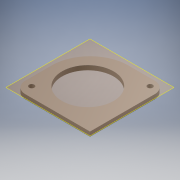
# Autodesk Inventor part: base
Saved by Autodesk Inventor 2016 (Build 200138000, 138)
## iProperties
Created: 2016-01-18
Part Number: base
Material: Generic
Document SubType Name: Modeling
Designer: Erwin Ried
Density: 1 g/cm^3
Appearance: Default
Author: Erwin Ried
Autodesk Inventor part; units mm, degrees
ref_plane "YZ Plane" through (0, 0, 0) normal (1, 0, 0) x (0, 1, 0)
ref_plane "XZ Plane" through (0, 0, 0) normal (0, 1, 0) x (-1, 0, 0)
ref_plane "XY Plane" through (0, 0, 0) normal (0, 0, 1) x (1, 0, 0)
ref_plane "Work Plane1" through (0, 0, 0) normal (0, 0, 1) x (1, 0, 0)
sketch "Sketch1" plane through (0, 0, 0) normal (0, 0, 1) x (1, 0, 0)
  line L0 (-5.1606, -11.1286) -> (-4.5083, -12.1241) projected
  line L1 (-4.5083, -12.1241) -> (-3.9263, -13.1603) projected
  line L2 (-3.9263, -13.1603) -> (-3.4128, -14.2404) projected
  line L3 (-3.4128, -14.2404) -> (-2.9734, -15.3534) projected
  line L4 (-2.9734, -15.3534) -> (-2.6124, -16.4922) projected
  line L5 (-2.6124, -16.4922) -> (-2.3286, -17.6568) projected
  line L6 (-2.3286, -17.6568) -> (-2.126, -18.8312) projected
  line L7 (-2.126, -18.8312) -> (-2.0043, -20.0161) projected
  line L8 (-2.0043, -20.0161) -> (-1.9632, -21.2132) projected
  line L9 (-2.0053, -22.4191) -> (-1.9632, -21.2132) projected
  line L10 (-2.1283, -23.6107) -> (-2.0053, -22.4191) projected
  line L11 (-2.3328, -24.7898) -> (-2.1283, -23.6107) projected
  line L12 (-2.6189, -25.957) -> (-2.3328, -24.7898) projected
  line L13 (-2.9818, -27.0966) -> (-2.6189, -25.957) projected
  line L14 (-3.4226, -28.2085) -> (-2.9818, -27.0966) projected
  line L15 (-3.9367, -29.2861) -> (-3.4226, -28.2085) projected
  line L16 (-4.5183, -30.3188) -> (-3.9367, -29.2861) projected
  line L17 (-5.169, -31.3097) -> (-4.5183, -30.3188) projected
  line L18 (-5.8865, -32.2545) -> (-5.169, -31.3097) projected
  line L19 (-6.6737, -33.1569) -> (-5.8865, -32.2545) projected
  line L20 (-7.5197, -34.0039) -> (-6.6737, -33.1569) projected
  line L21 (-8.4188, -34.7876) -> (-7.5197, -34.0039) projected
  line L22 (-9.3708, -35.5096) -> (-8.4188, -34.7876) projected
  line L23 (-10.3652, -36.1622) -> (-9.3708, -35.5096) projected
  line L24 (-11.405, -36.7472) -> (-10.3652, -36.1622) projected
  line L25 (-12.4791, -37.2591) -> (-11.405, -36.7472) projected
  line L26 (-13.5862, -37.6966) -> (-12.4791, -37.2591) projected
  line L27 (-14.722, -38.0586) -> (-13.5862, -37.6966) projected
  line L28 (-15.8764, -38.3415) -> (-14.722, -38.0586) projected
  line L29 (-17.0521, -38.5461) -> (-15.8764, -38.3415) projected
  line L30 (-18.2354, -38.67) -> (-17.0521, -38.5461) projected
  line L31 (-19.4276, -38.7129) -> (-18.2354, -38.67) projected
  line L32 (-20.6207, -38.6749) -> (-19.4276, -38.7129) projected
  line L33 (-21.8064, -38.5553) -> (-20.6207, -38.6749) projected
  line L34 (-22.9861, -38.3548) -> (-21.8064, -38.5553) projected
  line L35 (-24.1458, -38.0749) -> (-22.9861, -38.3548) projected
  line L36 (-25.2885, -37.7149) -> (-24.1458, -38.0749) projected
  line L37 (-26.4032, -37.2782) -> (-25.2885, -37.7149) projected
  line L38 (-27.4856, -36.7657) -> (-26.4032, -37.2782) projected
  line L39 (-28.534, -36.1787) -> (-27.4856, -36.7657) projected
  line L40 (-29.5366, -35.523) -> (-28.534, -36.1787) projected
  line L41 (-30.4963, -34.7966) -> (-29.5366, -35.523) projected
  line L42 (-31.4021, -34.0081) -> (-30.4963, -34.7966) projected
  line L43 (-32.2538, -33.1556) -> (-31.4021, -34.0081) projected
  line L44 (-33.0454, -32.2477) -> (-32.2538, -33.1556) projected
  line L45 (-33.7658, -31.2978) -> (-33.0454, -32.2477) projected
  line L46 (-34.4181, -30.3023) -> (-33.7658, -31.2978) projected
  line L47 (-35.0001, -29.2661) -> (-34.4181, -30.3023) projected
  line L48 (-35.5136, -28.186) -> (-35.0001, -29.2661) projected
  line L49 (-35.9529, -27.073) -> (-35.5136, -28.186) projected
  line L50 (-36.314, -25.9342) -> (-35.9529, -27.073) projected
  line L51 (-36.5978, -24.7695) -> (-36.314, -25.9342) projected
  line L52 (-36.8004, -23.5952) -> (-36.5978, -24.7695) projected
  line L53 (-36.9221, -22.4103) -> (-36.8004, -23.5952) projected
  line L54 (-36.9632, -21.2132) -> (-36.9221, -22.4103) projected
  line L55 (-36.9632, -21.2132) -> (-36.9211, -20.0072) projected
  line L56 (-36.9211, -20.0072) -> (-36.7981, -18.8157) projected
  line L57 (-36.7981, -18.8157) -> (-36.5936, -17.6366) projected
  line L58 (-36.5936, -17.6366) -> (-36.3075, -16.4694) projected
  line L59 (-36.3075, -16.4694) -> (-35.9446, -15.3298) projected
  line L60 (-35.9446, -15.3298) -> (-35.5038, -14.2179) projected
  line L61 (-35.5038, -14.2179) -> (-34.9897, -13.1403) projected
  line L62 (-34.9897, -13.1403) -> (-34.4081, -12.1076) projected
  line L63 (-34.4081, -12.1076) -> (-33.7574, -11.1167) projected
  line L64 (-33.7574, -11.1167) -> (-33.0399, -10.1719) projected
  line L65 (-33.0399, -10.1719) -> (-32.2527, -9.2695) projected
  line L66 (-32.2527, -9.2695) -> (-31.4066, -8.4225) projected
  line L67 (-31.4066, -8.4225) -> (-30.5076, -7.6388) projected
  line L68 (-30.5076, -7.6388) -> (-29.5556, -6.9168) projected
  line L69 (-29.5556, -6.9168) -> (-28.5612, -6.2641) projected
  line L70 (-28.5612, -6.2641) -> (-27.5214, -5.6792) projected
  line L71 (-27.5214, -5.6792) -> (-26.4473, -5.1673) projected
  line L72 (-26.4473, -5.1673) -> (-25.3402, -4.7298) projected
  line L73 (-25.3402, -4.7298) -> (-24.2044, -4.3678) projected
  line L74 (-24.2044, -4.3678) -> (-23.05, -4.0849) projected
  line L75 (-23.05, -4.0849) -> (-21.8743, -3.8803) projected
  line L76 (-21.8743, -3.8803) -> (-20.691, -3.7564) projected
  line L77 (-20.691, -3.7564) -> (-19.4988, -3.7135) projected
  line L78 (-19.4988, -3.7135) -> (-18.3057, -3.7515) projected
  line L79 (-18.3057, -3.7515) -> (-17.12, -3.8711) projected
  line L80 (-17.12, -3.8711) -> (-15.9403, -4.0716) projected
  line L81 (-15.9403, -4.0716) -> (-14.7806, -4.3515) projected
  line L82 (-14.7806, -4.3515) -> (-13.6379, -4.7115) projected
  line L83 (-13.6379, -4.7115) -> (-12.5232, -5.1482) projected
  line L84 (-12.5232, -5.1482) -> (-11.4408, -5.6607) projected
  line L85 (-11.4408, -5.6607) -> (-10.3924, -6.2477) projected
  line L86 (-10.3924, -6.2477) -> (-9.3899, -6.9034) projected
  line L87 (-9.3899, -6.9034) -> (-8.4301, -7.6298) projected
  line L88 (-8.4301, -7.6298) -> (-7.5242, -8.4183) projected
  line L89 (-7.5242, -8.4183) -> (-6.6726, -9.2707) projected
  line L90 (-6.6726, -9.2707) -> (-5.881, -10.1787) projected
  line L91 (-5.881, -10.1787) -> (-5.1606, -11.1286) projected
  line L92 (-36.9509, -39.6064) -> (-36.8705, -39.831) projected
  line L93 (-36.8705, -39.831) -> (-36.8223, -40.0632) projected
  line L94 (-36.8223, -40.0632) -> (-36.8051, -40.3051) projected
  line L95 (-36.8222, -40.5477) -> (-36.8051, -40.3051) projected
  line L96 (-36.8711, -40.7811) -> (-36.8222, -40.5477) projected
  line L97 (-36.9527, -41.0075) -> (-36.8711, -40.7811) projected
  line L98 (-37.0645, -41.2218) -> (-36.9527, -41.0075) projected
  line L99 (-37.2034, -41.4163) -> (-37.0645, -41.2218) projected
  line L100 (-37.3681, -41.5909) -> (-37.2034, -41.4163) projected
  line L101 (-37.5533, -41.7398) -> (-37.3681, -41.5909) projected
  line L102 (-37.7583, -41.8631) -> (-37.5533, -41.7398) projected
  line L103 (-37.9764, -41.9564) -> (-37.7583, -41.8631) projected
  line L104 (-38.2075, -42.0201) -> (-37.9764, -41.9564) projected
  line L105 (-38.4425, -42.0513) -> (-38.2075, -42.0201) projected
  line L106 (-38.6818, -42.0504) -> (-38.4425, -42.0513) projected
  line L107 (-38.9165, -42.0171) -> (-38.6818, -42.0504) projected
  line L108 (-39.1474, -41.9514) -> (-38.9165, -42.0171) projected
  line L109 (-39.3645, -41.8566) -> (-39.1474, -41.9514) projected
  line L110 (-39.5677, -41.7322) -> (-39.3645, -41.8566) projected
  line L111 (-39.7505, -41.5831) -> (-39.5677, -41.7322) projected
  line L112 (-39.9126, -41.4092) -> (-39.7505, -41.5831) projected
  line L113 (-40.0492, -41.216) -> (-39.9126, -41.4092) projected
  line L114 (-40.1593, -41.0037) -> (-40.0492, -41.216) projected
  line L115 (-40.2396, -40.7792) -> (-40.1593, -41.0037) projected
  line L116 (-40.2879, -40.547) -> (-40.2396, -40.7792) projected
  line L117 (-40.3051, -40.3051) -> (-40.2879, -40.547) projected
  line L118 (-40.3051, -40.3051) -> (-40.2879, -40.0625) projected
  line L119 (-40.2879, -40.0625) -> (-40.2391, -39.8291) projected
  line L120 (-40.2391, -39.8291) -> (-40.1575, -39.6027) projected
  line L121 (-40.1575, -39.6027) -> (-40.0457, -39.3884) projected
  line L122 (-40.0457, -39.3884) -> (-39.9067, -39.1939) projected
  line L123 (-39.9067, -39.1939) -> (-39.742, -39.0192) projected
  line L124 (-39.742, -39.0192) -> (-39.5569, -38.8704) projected
  line L125 (-39.5569, -38.8704) -> (-39.3518, -38.7471) projected
  line L126 (-39.3518, -38.7471) -> (-39.1338, -38.6538) projected
  line L127 (-39.1338, -38.6538) -> (-38.9026, -38.5901) projected
  line L128 (-38.9026, -38.5901) -> (-38.6677, -38.5588) projected
  line L129 (-38.6677, -38.5588) -> (-38.4284, -38.5598) projected
  line L130 (-38.4284, -38.5598) -> (-38.1936, -38.593) projected
  line L131 (-38.1936, -38.593) -> (-37.9627, -38.6587) projected
  line L132 (-37.9627, -38.6587) -> (-37.7456, -38.7536) projected
  line L133 (-37.7456, -38.7536) -> (-37.5425, -38.878) projected
  line L134 (-37.5425, -38.878) -> (-37.3596, -39.0271) projected
  line L135 (-37.3596, -39.0271) -> (-37.1975, -39.2009) projected
  line L136 (-37.1975, -39.2009) -> (-37.0609, -39.3941) projected
  line L137 (-37.0609, -39.3941) -> (-36.9509, -39.6064) projected
  line L138 (-40.1775, -46.0183) -> (-39.5312, -46.3784) projected
  line L139 (-39.5312, -46.3784) -> (-38.8571, -46.6766) projected
  line L140 (-38.8571, -46.6766) -> (-38.1554, -46.9119) projected
  line L141 (-38.1554, -46.9119) -> (-37.4366, -47.0815) projected
  line L142 (-37.4366, -47.0815) -> (-36.7069, -47.1834) projected
  line L143 (-36.7069, -47.1834) -> (-35.9632, -47.2184) projected
  line L144 (-35.9632, -47.2184) -> (-11.9632, -47.2184) projected
  line L145 (-11.9632, -47.2184) -> (-10.4632, -47.2184) projected
  line L146 (-10.4632, -47.2184) -> (6.5368, -47.2184) projected
  line L147 (6.5368, -47.2184) -> (8.0368, -47.2184) projected
  line L148 (8.0368, -47.2184) -> (8.0368, -3.2184) projected
  line L149 (8.0018, -2.4748) -> (8.0368, -3.2184) projected
  line L150 (7.8999, -1.745) -> (8.0018, -2.4748) projected
  line L151 (7.7304, -1.0263) -> (7.8999, -1.745) projected
  line L152 (7.495, -0.3246) -> (7.7304, -1.0263) projected
  line L153 (7.1969, 0.3495) -> (7.495, -0.3246) projected
  line L154 (6.8367, 0.9958) -> (7.1969, 0.3495) projected
  line L155 (6.4204, 1.6031) -> (6.8367, 0.9958) projected
  line L156 (5.9478, 2.1721) -> (6.4204, 1.6031) projected
  line L157 (5.4274, 2.6925) -> (5.9478, 2.1721) projected
  line L158 (4.8584, 3.1651) -> (5.4274, 2.6925) projected
  line L159 (4.2511, 3.5814) -> (4.8584, 3.1651) projected
  line L160 (3.6048, 3.9416) -> (4.2511, 3.5814) projected
  line L161 (2.9307, 4.2397) -> (3.6048, 3.9416) projected
  line L162 (2.229, 4.4751) -> (2.9307, 4.2397) projected
  line L163 (1.5103, 4.6447) -> (2.229, 4.4751) projected
  line L164 (0.7805, 4.7466) -> (1.5103, 4.6447) projected
  line L165 (0.0368, 4.7816) -> (0.7805, 4.7466) projected
  line L166 (-17.9632, 4.7816) -> (0.0368, 4.7816) projected
  line L167 (-19.4279, 4.7399) -> (-17.9632, 4.7816) projected
  line L168 (-20.8805, 4.6173) -> (-19.4279, 4.7399) projected
  line L169 (-22.322, 4.4136) -> (-20.8805, 4.6173) projected
  line L170 (-23.7547, 4.1281) -> (-22.322, 4.4136) projected
  line L171 (-25.1672, 3.7636) -> (-23.7547, 4.1281) projected
  line L172 (-26.5555, 3.3206) -> (-25.1672, 3.7636) projected
  line L173 (-27.9196, 2.7995) -> (-26.5555, 3.3206) projected
  line L174 (-29.2482, 2.2048) -> (-27.9196, 2.7995) projected
  line L175 (-30.5443, 1.5347) -> (-29.2482, 2.2048) projected
  line L176 (-31.8002, 0.7938) -> (-30.5443, 1.5347) projected
  line L177 (-33.0104, -0.0153) -> (-31.8002, 0.7938) projected
  line L178 (-34.1764, -0.893) -> (-33.0104, -0.0153) projected
  line L179 (-35.2883, -1.8318) -> (-34.1764, -0.893) projected
  line L180 (-36.3477, -2.8337) -> (-35.2883, -1.8318) projected
  line L181 (-37.3497, -3.8932) -> (-36.3477, -2.8337) projected
  line L182 (-38.2885, -5.0051) -> (-37.3497, -3.8932) projected
  line L183 (-39.1662, -6.1711) -> (-38.2885, -5.0051) projected
  line L184 (-39.9753, -7.3813) -> (-39.1662, -6.1711) projected
  line L185 (-40.7162, -8.6371) -> (-39.9753, -7.3813) projected
  line L186 (-41.3863, -9.9332) -> (-40.7162, -8.6371) projected
  line L187 (-41.9811, -11.2619) -> (-41.3863, -9.9332) projected
  line L188 (-42.5022, -12.626) -> (-41.9811, -11.2619) projected
  line L189 (-42.9452, -14.0143) -> (-42.5022, -12.626) projected
  line L190 (-43.3097, -15.4268) -> (-42.9452, -14.0143) projected
  line L191 (-43.5951, -16.8595) -> (-43.3097, -15.4268) projected
  line L192 (-43.7989, -18.3011) -> (-43.5951, -16.8595) projected
  line L193 (-43.9215, -19.7537) -> (-43.7989, -18.3011) projected
  line L194 (-43.9632, -21.2184) -> (-43.9215, -19.7537) projected
  line L195 (-43.9632, -39.2184) -> (-43.9632, -21.2184) projected
  line L196 (-43.9632, -39.2184) -> (-43.9282, -39.962) projected
  line L197 (-43.9282, -39.962) -> (-43.8263, -40.6918) projected
  line L198 (-43.8263, -40.6918) -> (-43.6568, -41.4105) projected
  line L199 (-43.6568, -41.4105) -> (-43.4214, -42.1122) projected
  line L200 (-43.4214, -42.1122) -> (-43.1233, -42.7863) projected
  line L201 (-43.1233, -42.7863) -> (-42.7631, -43.4326) projected
  line L202 (-42.7631, -43.4326) -> (-42.3468, -44.0399) projected
  line L203 (-42.3468, -44.0399) -> (-41.8742, -44.6089) projected
  line L204 (-41.8742, -44.6089) -> (-41.3538, -45.1293) projected
  line L205 (-41.3538, -45.1293) -> (-40.7848, -45.6019) projected
  line L206 (-40.7848, -45.6019) -> (-40.1775, -46.0183) projected
  line L207 (0, 0) -> (0.0172, 0.2426) projected
  line L208 (0.0172, 0.2426) -> (0.066, 0.476) projected
  line L209 (0.066, 0.476) -> (0.1476, 0.7024) projected
  line L210 (0.1476, 0.7024) -> (0.2594, 0.9167) projected
  line L211 (0.2594, 0.9167) -> (0.3983, 1.1112) projected
  line L212 (0.3983, 1.1112) -> (0.5631, 1.2858) projected
  line L213 (0.5631, 1.2858) -> (0.7482, 1.4347) projected
  line L214 (0.7482, 1.4347) -> (0.9532, 1.558) projected
  line L215 (0.9532, 1.558) -> (1.1713, 1.6513) projected
  line L216 (1.1713, 1.6513) -> (1.4025, 1.715) projected
  line L217 (1.4025, 1.715) -> (1.6374, 1.7462) projected
  line L218 (1.6374, 1.7462) -> (1.8767, 1.7453) projected
  line L219 (1.8767, 1.7453) -> (2.1115, 1.7121) projected
  line L220 (2.1115, 1.7121) -> (2.3424, 1.6464) projected
  line L221 (2.3424, 1.6464) -> (2.5595, 1.5515) projected
  line L222 (2.5595, 1.5515) -> (2.7626, 1.4271) projected
  line L223 (2.7626, 1.4271) -> (2.9455, 1.278) projected
  line L224 (2.9455, 1.278) -> (3.1075, 1.1041) projected
  line L225 (3.1075, 1.1041) -> (3.2441, 0.911) projected
  line L226 (3.2441, 0.911) -> (3.3542, 0.6986) projected
  line L227 (3.3542, 0.6986) -> (3.4345, 0.4741) projected
  line L228 (3.4345, 0.4741) -> (3.4828, 0.2419) projected
  line L229 (3.4828, 0.2419) -> (3.5, 0) projected
  line L230 (3.4828, -0.2426) -> (3.5, 0) projected
  line L231 (3.434, -0.476) -> (3.4828, -0.2426) projected
  line L232 (3.3524, -0.7024) -> (3.434, -0.476) projected
  line L233 (3.2406, -0.9167) -> (3.3524, -0.7024) projected
  line L234 (3.1017, -1.1112) -> (3.2406, -0.9167) projected
  line L235 (2.9369, -1.2858) -> (3.1017, -1.1112) projected
  line L236 (2.7518, -1.4347) -> (2.9369, -1.2858) projected
  line L237 (2.5468, -1.558) -> (2.7518, -1.4347) projected
  line L238 (2.3287, -1.6513) -> (2.5468, -1.558) projected
  line L239 (2.0976, -1.715) -> (2.3287, -1.6513) projected
  line L240 (1.8626, -1.7462) -> (2.0976, -1.715) projected
  line L241 (1.6233, -1.7453) -> (1.8626, -1.7462) projected
  line L242 (1.3885, -1.7121) -> (1.6233, -1.7453) projected
  line L243 (1.1576, -1.6464) -> (1.3885, -1.7121) projected
  line L244 (0.9405, -1.5515) -> (1.1576, -1.6464) projected
  line L245 (0.7374, -1.4271) -> (0.9405, -1.5515) projected
  line L246 (0.5545, -1.278) -> (0.7374, -1.4271) projected
  line L247 (0.3925, -1.1041) -> (0.5545, -1.278) projected
  line L248 (0.2559, -0.9109) -> (0.3925, -1.1041) projected
  line L249 (0.1458, -0.6986) -> (0.2559, -0.9109) projected
  line L250 (0.0655, -0.4741) -> (0.1458, -0.6986) projected
  line L251 (0.0172, -0.2419) -> (0.0655, -0.4741) projected
  line L252 (0, 0) -> (0.0172, -0.2419) projected
  line L253 (-5.1606, -11.1286) -> (-4.5083, -12.1241) projected
  line L254 (-4.5083, -12.1241) -> (-3.9263, -13.1603) projected
  line L255 (-3.9263, -13.1603) -> (-3.4128, -14.2404) projected
  line L256 (-3.4128, -14.2404) -> (-2.9734, -15.3534) projected
  line L257 (-2.9734, -15.3534) -> (-2.6124, -16.4922) projected
  line L258 (-2.6124, -16.4922) -> (-2.3286, -17.6568) projected
  line L259 (-2.3286, -17.6568) -> (-2.126, -18.8312) projected
  line L260 (-2.126, -18.8312) -> (-2.0043, -20.0161) projected
  line L261 (-2.0043, -20.0161) -> (-1.9632, -21.2132) projected
  line L262 (-2.0053, -22.4191) -> (-1.9632, -21.2132) projected
  line L263 (-2.1283, -23.6107) -> (-2.0053, -22.4191) projected
  line L264 (-2.3328, -24.7898) -> (-2.1283, -23.6107) projected
  line L265 (-2.6189, -25.957) -> (-2.3328, -24.7898) projected
  line L266 (-2.9818, -27.0966) -> (-2.6189, -25.957) projected
  line L267 (-3.4226, -28.2085) -> (-2.9818, -27.0966) projected
  line L268 (-3.9367, -29.2861) -> (-3.4226, -28.2085) projected
  line L269 (-4.5183, -30.3188) -> (-3.9367, -29.2861) projected
  line L270 (-5.169, -31.3097) -> (-4.5183, -30.3188) projected
  line L271 (-5.8865, -32.2545) -> (-5.169, -31.3097) projected
  line L272 (-6.6737, -33.1569) -> (-5.8865, -32.2545) projected
  line L273 (-7.5197, -34.0039) -> (-6.6737, -33.1569) projected
  line L274 (-8.4188, -34.7876) -> (-7.5197, -34.0039) projected
  line L275 (-9.3708, -35.5096) -> (-8.4188, -34.7876) projected
  line L276 (-10.3652, -36.1622) -> (-9.3708, -35.5096) projected
  line L277 (-11.405, -36.7472) -> (-10.3652, -36.1622) projected
  line L278 (-12.4791, -37.2591) -> (-11.405, -36.7472) projected
  line L279 (-13.5862, -37.6966) -> (-12.4791, -37.2591) projected
  line L280 (-14.722, -38.0586) -> (-13.5862, -37.6966) projected
  line L281 (-15.8764, -38.3415) -> (-14.722, -38.0586) projected
  line L282 (-17.0521, -38.5461) -> (-15.8764, -38.3415) projected
  line L283 (-18.2354, -38.67) -> (-17.0521, -38.5461) projected
  line L284 (-19.4276, -38.7129) -> (-18.2354, -38.67) projected
  line L285 (-20.6207, -38.6749) -> (-19.4276, -38.7129) projected
  line L286 (-21.8064, -38.5553) -> (-20.6207, -38.6749) projected
  line L287 (-22.9861, -38.3548) -> (-21.8064, -38.5553) projected
  line L288 (-24.1458, -38.0749) -> (-22.9861, -38.3548) projected
  line L289 (-25.2885, -37.7149) -> (-24.1458, -38.0749) projected
  line L290 (-26.4032, -37.2782) -> (-25.2885, -37.7149) projected
  line L291 (-27.4856, -36.7657) -> (-26.4032, -37.2782) projected
  line L292 (-28.534, -36.1787) -> (-27.4856, -36.7657) projected
  line L293 (-29.5366, -35.523) -> (-28.534, -36.1787) projected
  line L294 (-30.4963, -34.7966) -> (-29.5366, -35.523) projected
  line L295 (-31.4021, -34.0081) -> (-30.4963, -34.7966) projected
  line L296 (-32.2538, -33.1556) -> (-31.4021, -34.0081) projected
  line L297 (-33.0454, -32.2477) -> (-32.2538, -33.1556) projected
  line L298 (-33.7658, -31.2978) -> (-33.0454, -32.2477) projected
  line L299 (-34.4181, -30.3023) -> (-33.7658, -31.2978) projected
  line L300 (-35.0001, -29.2661) -> (-34.4181, -30.3023) projected
  line L301 (-35.5136, -28.186) -> (-35.0001, -29.2661) projected
  line L302 (-35.9529, -27.073) -> (-35.5136, -28.186) projected
  line L303 (-36.314, -25.9342) -> (-35.9529, -27.073) projected
  line L304 (-36.5978, -24.7695) -> (-36.314, -25.9342) projected
  line L305 (-36.8004, -23.5952) -> (-36.5978, -24.7695) projected
  line L306 (-36.9221, -22.4103) -> (-36.8004, -23.5952) projected
  line L307 (-36.9632, -21.2132) -> (-36.9221, -22.4103) projected
  line L308 (-36.9632, -21.2132) -> (-36.9211, -20.0072) projected
  line L309 (-36.9211, -20.0072) -> (-36.7981, -18.8157) projected
  line L310 (-36.7981, -18.8157) -> (-36.5936, -17.6366) projected
  line L311 (-36.5936, -17.6366) -> (-36.3075, -16.4694) projected
  line L312 (-36.3075, -16.4694) -> (-35.9446, -15.3298) projected
  line L313 (-35.9446, -15.3298) -> (-35.5038, -14.2179) projected
  line L314 (-35.5038, -14.2179) -> (-34.9897, -13.1403) projected
  line L315 (-34.9897, -13.1403) -> (-34.4081, -12.1076) projected
  line L316 (-34.4081, -12.1076) -> (-33.7574, -11.1167) projected
  line L317 (-33.7574, -11.1167) -> (-33.0399, -10.1719) projected
  line L318 (-33.0399, -10.1719) -> (-32.2527, -9.2695) projected
  line L319 (-32.2527, -9.2695) -> (-31.4066, -8.4225) projected
  line L320 (-31.4066, -8.4225) -> (-30.5076, -7.6388) projected
  line L321 (-30.5076, -7.6388) -> (-29.5556, -6.9168) projected
  line L322 (-29.5556, -6.9168) -> (-28.5612, -6.2641) projected
  line L323 (-28.5612, -6.2641) -> (-27.5214, -5.6792) projected
  line L324 (-27.5214, -5.6792) -> (-26.4473, -5.1673) projected
  line L325 (-26.4473, -5.1673) -> (-25.3402, -4.7298) projected
  line L326 (-25.3402, -4.7298) -> (-24.2044, -4.3678) projected
  line L327 (-24.2044, -4.3678) -> (-23.05, -4.0849) projected
  line L328 (-23.05, -4.0849) -> (-21.8743, -3.8803) projected
  line L329 (-21.8743, -3.8803) -> (-20.691, -3.7564) projected
  line L330 (-20.691, -3.7564) -> (-19.4988, -3.7135) projected
  line L331 (-19.4988, -3.7135) -> (-18.3057, -3.7515) projected
  line L332 (-18.3057, -3.7515) -> (-17.12, -3.8711) projected
  line L333 (-17.12, -3.8711) -> (-15.9403, -4.0716) projected
  line L334 (-15.9403, -4.0716) -> (-14.7806, -4.3515) projected
  line L335 (-14.7806, -4.3515) -> (-13.6379, -4.7115) projected
  line L336 (-13.6379, -4.7115) -> (-12.5232, -5.1482) projected
  line L337 (-12.5232, -5.1482) -> (-11.4408, -5.6607) projected
  line L338 (-11.4408, -5.6607) -> (-10.3924, -6.2477) projected
  line L339 (-10.3924, -6.2477) -> (-9.3899, -6.9034) projected
  line L340 (-9.3899, -6.9034) -> (-8.4301, -7.6298) projected
  line L341 (-8.4301, -7.6298) -> (-7.5242, -8.4183) projected
  line L342 (-7.5242, -8.4183) -> (-6.6726, -9.2707) projected
  line L343 (-6.6726, -9.2707) -> (-5.881, -10.1787) projected
  line L344 (-5.881, -10.1787) -> (-5.1606, -11.1286) projected
  line L345 (-36.9509, -39.6064) -> (-36.8705, -39.831) projected
  line L346 (-36.8705, -39.831) -> (-36.8223, -40.0632) projected
  line L347 (-36.8223, -40.0632) -> (-36.8051, -40.3051) projected
  line L348 (-36.8222, -40.5477) -> (-36.8051, -40.3051) projected
  line L349 (-36.8711, -40.7811) -> (-36.8222, -40.5477) projected
  line L350 (-36.9527, -41.0075) -> (-36.8711, -40.7811) projected
  line L351 (-37.0645, -41.2218) -> (-36.9527, -41.0075) projected
  line L352 (-37.2034, -41.4163) -> (-37.0645, -41.2218) projected
  line L353 (-37.3681, -41.5909) -> (-37.2034, -41.4163) projected
  line L354 (-37.5533, -41.7398) -> (-37.3681, -41.5909) projected
  line L355 (-37.7583, -41.8631) -> (-37.5533, -41.7398) projected
  line L356 (-37.9764, -41.9564) -> (-37.7583, -41.8631) projected
  line L357 (-38.2075, -42.0201) -> (-37.9764, -41.9564) projected
  line L358 (-38.4425, -42.0513) -> (-38.2075, -42.0201) projected
  line L359 (-38.6818, -42.0504) -> (-38.4425, -42.0513) projected
  line L360 (-38.9165, -42.0171) -> (-38.6818, -42.0504) projected
  line L361 (-39.1474, -41.9514) -> (-38.9165, -42.0171) projected
  line L362 (-39.3645, -41.8566) -> (-39.1474, -41.9514) projected
  line L363 (-39.5677, -41.7322) -> (-39.3645, -41.8566) projected
  line L364 (-39.7505, -41.5831) -> (-39.5677, -41.7322) projected
  line L365 (-39.9126, -41.4092) -> (-39.7505, -41.5831) projected
  line L366 (-40.0492, -41.216) -> (-39.9126, -41.4092) projected
  line L367 (-40.1593, -41.0037) -> (-40.0492, -41.216) projected
  line L368 (-40.2396, -40.7792) -> (-40.1593, -41.0037) projected
  line L369 (-40.2879, -40.547) -> (-40.2396, -40.7792) projected
  line L370 (-40.3051, -40.3051) -> (-40.2879, -40.547) projected
  line L371 (-40.3051, -40.3051) -> (-40.2879, -40.0625) projected
  line L372 (-40.2879, -40.0625) -> (-40.2391, -39.8291) projected
  line L373 (-40.2391, -39.8291) -> (-40.1575, -39.6027) projected
  line L374 (-40.1575, -39.6027) -> (-40.0457, -39.3884) projected
  line L375 (-40.0457, -39.3884) -> (-39.9067, -39.1939) projected
  line L376 (-39.9067, -39.1939) -> (-39.742, -39.0192) projected
  line L377 (-39.742, -39.0192) -> (-39.5569, -38.8704) projected
  line L378 (-39.5569, -38.8704) -> (-39.3518, -38.7471) projected
  line L379 (-39.3518, -38.7471) -> (-39.1338, -38.6538) projected
  line L380 (-39.1338, -38.6538) -> (-38.9026, -38.5901) projected
  line L381 (-38.9026, -38.5901) -> (-38.6677, -38.5588) projected
  line L382 (-38.6677, -38.5588) -> (-38.4284, -38.5598) projected
  line L383 (-38.4284, -38.5598) -> (-38.1936, -38.593) projected
  line L384 (-38.1936, -38.593) -> (-37.9627, -38.6587) projected
  line L385 (-37.9627, -38.6587) -> (-37.7456, -38.7536) projected
  line L386 (-37.7456, -38.7536) -> (-37.5425, -38.878) projected
  line L387 (-37.5425, -38.878) -> (-37.3596, -39.0271) projected
  line L388 (-37.3596, -39.0271) -> (-37.1975, -39.2009) projected
  line L389 (-37.1975, -39.2009) -> (-37.0609, -39.3941) projected
  line L390 (-37.0609, -39.3941) -> (-36.9509, -39.6064) projected
  line L391 (-40.1775, -46.0183) -> (-39.5312, -46.3784) projected
  line L392 (-39.5312, -46.3784) -> (-38.8571, -46.6766) projected
  line L393 (-38.8571, -46.6766) -> (-38.1554, -46.9119) projected
  line L394 (-38.1554, -46.9119) -> (-37.4366, -47.0815) projected
  line L395 (-37.4366, -47.0815) -> (-36.7069, -47.1834) projected
  line L396 (-36.7069, -47.1834) -> (-35.9632, -47.2184) projected
  line L397 (-35.9632, -47.2184) -> (-11.9632, -47.2184) projected
  line L398 (-11.9632, -47.2184) -> (-10.4632, -47.2184) projected
  line L399 (-10.4632, -47.2184) -> (6.5368, -47.2184) projected
  line L400 (6.5368, -47.2184) -> (8.0368, -47.2184) projected
  line L401 (8.0368, -47.2184) -> (8.0368, -3.2184) projected
  line L402 (8.0018, -2.4748) -> (8.0368, -3.2184) projected
  line L403 (7.8999, -1.745) -> (8.0018, -2.4748) projected
  line L404 (7.7304, -1.0263) -> (7.8999, -1.745) projected
  line L405 (7.495, -0.3246) -> (7.7304, -1.0263) projected
  line L406 (7.1969, 0.3495) -> (7.495, -0.3246) projected
  line L407 (6.8367, 0.9958) -> (7.1969, 0.3495) projected
  line L408 (6.4204, 1.6031) -> (6.8367, 0.9958) projected
  line L409 (5.9478, 2.1721) -> (6.4204, 1.6031) projected
  line L410 (5.4274, 2.6925) -> (5.9478, 2.1721) projected
  line L411 (4.8584, 3.1651) -> (5.4274, 2.6925) projected
  line L412 (4.2511, 3.5814) -> (4.8584, 3.1651) projected
  line L413 (3.6048, 3.9416) -> (4.2511, 3.5814) projected
  line L414 (2.9307, 4.2397) -> (3.6048, 3.9416) projected
  line L415 (2.229, 4.4751) -> (2.9307, 4.2397) projected
  line L416 (1.5103, 4.6447) -> (2.229, 4.4751) projected
  line L417 (0.7805, 4.7466) -> (1.5103, 4.6447) projected
  line L418 (0.0368, 4.7816) -> (0.7805, 4.7466) projected
  line L419 (-17.9632, 4.7816) -> (0.0368, 4.7816) projected
  line L420 (-19.4279, 4.7399) -> (-17.9632, 4.7816) projected
  line L421 (-20.8805, 4.6173) -> (-19.4279, 4.7399) projected
  line L422 (-22.322, 4.4136) -> (-20.8805, 4.6173) projected
  line L423 (-23.7547, 4.1281) -> (-22.322, 4.4136) projected
  line L424 (-25.1672, 3.7636) -> (-23.7547, 4.1281) projected
  line L425 (-26.5555, 3.3206) -> (-25.1672, 3.7636) projected
  line L426 (-27.9196, 2.7995) -> (-26.5555, 3.3206) projected
  line L427 (-29.2482, 2.2048) -> (-27.9196, 2.7995) projected
  line L428 (-30.5443, 1.5347) -> (-29.2482, 2.2048) projected
  line L429 (-31.8002, 0.7938) -> (-30.5443, 1.5347) projected
  line L430 (-33.0104, -0.0153) -> (-31.8002, 0.7938) projected
  line L431 (-34.1764, -0.893) -> (-33.0104, -0.0153) projected
  line L432 (-35.2883, -1.8318) -> (-34.1764, -0.893) projected
  line L433 (-36.3477, -2.8337) -> (-35.2883, -1.8318) projected
  line L434 (-37.3497, -3.8932) -> (-36.3477, -2.8337) projected
  line L435 (-38.2885, -5.0051) -> (-37.3497, -3.8932) projected
  line L436 (-39.1662, -6.1711) -> (-38.2885, -5.0051) projected
  line L437 (-39.9753, -7.3813) -> (-39.1662, -6.1711) projected
  line L438 (-40.7162, -8.6371) -> (-39.9753, -7.3813) projected
  line L439 (-41.3863, -9.9332) -> (-40.7162, -8.6371) projected
  line L440 (-41.9811, -11.2619) -> (-41.3863, -9.9332) projected
  line L441 (-42.5022, -12.626) -> (-41.9811, -11.2619) projected
  line L442 (-42.9452, -14.0143) -> (-42.5022, -12.626) projected
  line L443 (-43.3097, -15.4268) -> (-42.9452, -14.0143) projected
  line L444 (-43.5951, -16.8595) -> (-43.3097, -15.4268) projected
  line L445 (-43.7989, -18.3011) -> (-43.5951, -16.8595) projected
  line L446 (-43.9215, -19.7537) -> (-43.7989, -18.3011) projected
  line L447 (-43.9632, -21.2184) -> (-43.9215, -19.7537) projected
  line L448 (-43.9632, -39.2184) -> (-43.9632, -21.2184) projected
  line L449 (-43.9632, -39.2184) -> (-43.9282, -39.962) projected
  line L450 (-43.9282, -39.962) -> (-43.8263, -40.6918) projected
  line L451 (-43.8263, -40.6918) -> (-43.6568, -41.4105) projected
  line L452 (-43.6568, -41.4105) -> (-43.4214, -42.1122) projected
  line L453 (-43.4214, -42.1122) -> (-43.1233, -42.7863) projected
  line L454 (-43.1233, -42.7863) -> (-42.7631, -43.4326) projected
  line L455 (-42.7631, -43.4326) -> (-42.3468, -44.0399) projected
  line L456 (-42.3468, -44.0399) -> (-41.8742, -44.6089) projected
  line L457 (-41.8742, -44.6089) -> (-41.3538, -45.1293) projected
  line L458 (-41.3538, -45.1293) -> (-40.7848, -45.6019) projected
  line L459 (-40.7848, -45.6019) -> (-40.1775, -46.0183) projected
  line L460 (0, 0) -> (0.0172, 0.2426) projected
  line L461 (0.0172, 0.2426) -> (0.066, 0.476) projected
  line L462 (0.066, 0.476) -> (0.1476, 0.7024) projected
  line L463 (0.1476, 0.7024) -> (0.2594, 0.9167) projected
  line L464 (0.2594, 0.9167) -> (0.3983, 1.1112) projected
  line L465 (0.3983, 1.1112) -> (0.5631, 1.2858) projected
  line L466 (0.5631, 1.2858) -> (0.7482, 1.4347) projected
  line L467 (0.7482, 1.4347) -> (0.9532, 1.558) projected
  line L468 (0.9532, 1.558) -> (1.1713, 1.6513) projected
  line L469 (1.1713, 1.6513) -> (1.4025, 1.715) projected
  line L470 (1.4025, 1.715) -> (1.6374, 1.7462) projected
  line L471 (1.6374, 1.7462) -> (1.8767, 1.7453) projected
  line L472 (1.8767, 1.7453) -> (2.1115, 1.7121) projected
  line L473 (2.1115, 1.7121) -> (2.3424, 1.6464) projected
  line L474 (2.3424, 1.6464) -> (2.5595, 1.5515) projected
  line L475 (2.5595, 1.5515) -> (2.7626, 1.4271) projected
  line L476 (2.7626, 1.4271) -> (2.9455, 1.278) projected
  line L477 (2.9455, 1.278) -> (3.1075, 1.1041) projected
  line L478 (3.1075, 1.1041) -> (3.2441, 0.911) projected
  line L479 (3.2441, 0.911) -> (3.3542, 0.6986) projected
  line L480 (3.3542, 0.6986) -> (3.4345, 0.4741) projected
  line L481 (3.4345, 0.4741) -> (3.4828, 0.2419) projected
  line L482 (3.4828, 0.2419) -> (3.5, 0) projected
  line L483 (3.4828, -0.2426) -> (3.5, 0) projected
  line L484 (3.434, -0.476) -> (3.4828, -0.2426) projected
  line L485 (3.3524, -0.7024) -> (3.434, -0.476) projected
  line L486 (3.2406, -0.9167) -> (3.3524, -0.7024) projected
  line L487 (3.1017, -1.1112) -> (3.2406, -0.9167) projected
  line L488 (2.9369, -1.2858) -> (3.1017, -1.1112) projected
  line L489 (2.7518, -1.4347) -> (2.9369, -1.2858) projected
  line L490 (2.5468, -1.558) -> (2.7518, -1.4347) projected
  line L491 (2.3287, -1.6513) -> (2.5468, -1.558) projected
  line L492 (2.0976, -1.715) -> (2.3287, -1.6513) projected
  line L493 (1.8626, -1.7462) -> (2.0976, -1.715) projected
  line L494 (1.6233, -1.7453) -> (1.8626, -1.7462) projected
  line L495 (1.3885, -1.7121) -> (1.6233, -1.7453) projected
  line L496 (1.1576, -1.6464) -> (1.3885, -1.7121) projected
  line L497 (0.9405, -1.5515) -> (1.1576, -1.6464) projected
  line L498 (0.7374, -1.4271) -> (0.9405, -1.5515) projected
  line L499 (0.5545, -1.278) -> (0.7374, -1.4271) projected
  line L500 (0.3925, -1.1041) -> (0.5545, -1.278) projected
  line L501 (0.2559, -0.9109) -> (0.3925, -1.1041) projected
  line L502 (0.1458, -0.6986) -> (0.2559, -0.9109) projected
  line L503 (0.0655, -0.4741) -> (0.1458, -0.6986) projected
  line L504 (0.0172, -0.2419) -> (0.0655, -0.4741) projected
  line L505 (0, 0) -> (0.0172, -0.2419) projected
extrude "Extrusion1" add sketch "Sketch1" against normal blind 3
body "Solid1"
